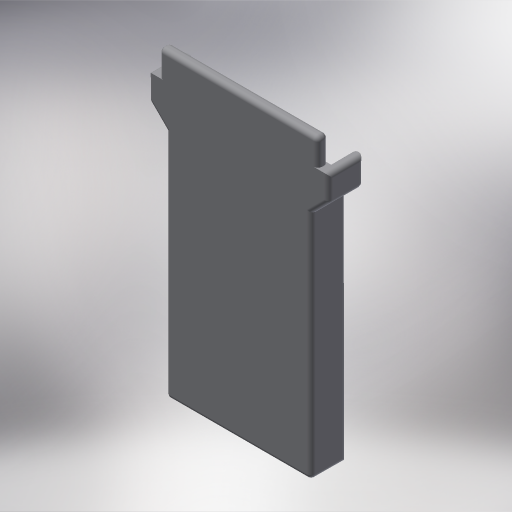
# Autodesk Inventor part: cover_02 wider
Saved by Autodesk Inventor 2023 (Build 270158000, 158)
## iProperties
Created: 2013-11-30
Part Number: cover_02 wider
Material: Generic
Document SubType Name: Modeling
Designer: Labadmin
Density: 1 g/cm^3
Appearance: Default
Author: Labadmin
Autodesk Inventor part; units mm, degrees
ref_plane "YZ Plane" through (0, 0, 0) normal (1, 0, 0) x (0, 1, 0)
ref_plane "XZ Plane" through (0, 0, 0) normal (0, 1, 0) x (-1, 0, 0)
ref_plane "XY Plane" through (0, 0, 0) normal (0, 0, 1) x (1, 0, 0)
sketch "Sketch1" plane through (0, 0, 0) normal (0, 0, 1) x (1, 0, 0)
  line L0 (-40.005, 0) -> (40.005, 0) projected
  line L1 (0, -129.54) -> (0, 21.59) projected
  line L2 (-28.575, 0) -> (28.575, 0)
  line L3 (28.575, -18.542) -> (28.575, 0)
  line L4 (28.575, -18.542) -> (22.352, -24.765)
  line L5 (22.352, -24.765) -> (22.352, -107.95)
  line L6 (22.352, -107.95) -> (-22.352, -107.95)
  line L7 (-22.352, -107.95) -> (-22.352, -24.765)
  line L8 (-22.352, -24.765) -> (-28.575, -18.542)
  line L9 (-28.575, -18.542) -> (-28.575, 0)
  point P0 (0, 0)
  point P1 (0, -107.95)
  dimension "d0" = 57.15
  dimension "d1" = 107.95
  dimension "d3" = 44.704
  dimension "d4" = 135
  dimension "d20" = 83.185
  constraints: 16 end point, 4 perpendicular, 2 horizontal alignment, 2 midpoint, 2 point on line, 1 parallel
  measures "d0" distance between parallel lines of L3 L9
  measures "d1" distance between parallel lines of L6 L2
  measures "d3" distance of L5.end L6.end
  measures "d4" angle of L8 L9
  measures "d20" distance of L6.end L7.end
extrude "Extrusion1" add sketch "Sketch1" against normal blind 3.81
sketch "Sketch2" plane through (0, 0, 0) normal (0, 0, 1) x (1, 0, 0)
  line L0 (-22.352, -107.95) -> (22.352, -107.95) projected
  line L1 (22.352, -107.95) -> (22.352, -24.765) projected
  line L2 (22.352, -24.765) -> (28.575, -18.542) projected
  line L3 (28.575, -18.542) -> (28.575, 0) projected
  line L4 (28.575, 0) -> (-28.575, 0) projected
  line L5 (-28.575, 0) -> (-28.575, -18.542) projected
  line L6 (-28.575, -18.542) -> (-22.352, -24.765) projected
  line L7 (-22.352, -24.765) -> (-22.352, -107.95) projected
  line L8 (26.162, -24.765) -> (26.162, -107.95)
  line L9 (-26.162, -107.95) -> (-26.162, -24.765)
  line L10 (-26.162, -24.765) -> (-32.385, -18.542)
  line L11 (-32.385, -18.542) -> (-32.385, -9.525)
  line L12 (32.385, -9.525) -> (32.385, -18.542)
  line L13 (32.385, -18.542) -> (26.162, -24.765)
  line L14 (22.352, -107.95) -> (26.162, -107.95)
  line L15 (-22.352, -107.95) -> (-26.162, -107.95)
  line L16 (-32.385, -9.525) -> (-28.575, -9.525)
  line L17 (-28.575, -9.525) -> (-28.575, -18.542)
  line L18 (32.385, -9.525) -> (28.575, -9.525)
  line L19 (28.575, -9.525) -> (28.575, -18.542)
  point P0 (0, 0)
  dimension "d9" = 3.81
  dimension "d10" = 3.81
  dimension "d16" = 9.525
  dimension "d17" = 3.81
  dimension "d18" = 3.81
  constraints: 24 end point, 5 perpendicular, 3 horizontal alignment, 3 parallel, 2 collinear, 2 point on line
  measures "d9" distance of L0.start L9.start
  measures "d10" distance of L0.end L8.end
  measures "d16" distance between parallel lines of L16 L4
  measures "d17" distance between parallel lines of L17 L11
  measures "d18" distance between parallel lines of L19 L12
extrude "Extrusion2" add sketch "Sketch2" against normal blind 12.7 contours L15 L9 L10 L11 L16 L5 L6 L7 | L1 L2 L3 L18 L12 L13 L8 L14
fillet "Fillet1" radius 3.175 2 edges at (22.352, -24.765, -8.255) (-22.352, -24.765, -8.255)
fillet "Fillet2" radius 1.5875 13 edges at (-22.5937, -24.8651, -12.7) (-25.9285, -21.1885, -12.7) (-22.352, -67.0151, -12.7) (22.5937, -24.8651, -12.7) (25.9285, -21.1885, -12.7) (22.352, -67.0151, -12.7) (-28.575, -14.0335, -12.7) (28.575, -14.0335, -12.7) (22.352, -107.95, -8.255) (-22.352, -107.95, -8.255) (0, -107.95, -3.81) (-28.575, -9.525, -8.255) (28.575, -9.525, -8.255)
fillet "Fillet3" radius 1.5875 18 edges at (-26.162, -107.95, -6.35) (-26.162, -66.3575, -12.7) (-26.162, -66.3575, 0) (-29.2735, -21.6535, -12.7) (-29.2735, -21.6535, 0) (-32.385, -18.542, -6.35) (-32.385, -14.0335, 0) (-32.385, -14.0335, -12.7) (-32.385, -9.525, -6.35) (26.162, -107.95, -6.35) (26.162, -66.3575, 0) (26.162, -66.3575, -12.7) (29.2735, -21.6535, 0) (29.2735, -21.6535, -12.7) (32.385, -18.542, -6.35) (32.385, -14.0335, -12.7) (32.385, -14.0335, 0) (32.385, -9.525, -6.35)
fillet "Fillet4" radius 1.5875 1 edges at (0, -107.95, 0)
fillet "Fillet5" radius 1.5875 8 edges at (28.575, 0, -1.905) (0, 0, 0) (-28.575, 0, -1.905) (0, 0, -3.81) (-28.575, -4.7625, -3.81) (28.575, -4.7625, -3.81) (28.575, -4.7625, 0) (-28.575, -4.7625, 0)
equation "\"d9\" = d7"
equation "\"d10\" = d7"
equation "\"d18\" = d17"
equation "\"d7\" = 3.81"
body "Solid1"
